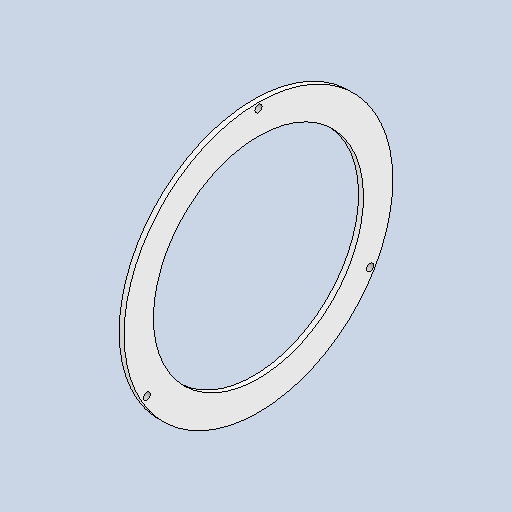
# Autodesk Inventor part: joint3_base_cover
Saved by Autodesk Inventor 2025.3 (Build 293356030, 356C)
## iProperties
Created: 2025-11-21
Part Number: joint3_base_cover
Material: PLA filament
Document SubType Name: Modeling
Designer: MSI
Mass: 17.2219 g
Surface Area: 134.924 cm^2
Volume: 14.3516 cm^3
Density: 1.2 g/cm^3
Appearance: 일반
Author: MSI
Autodesk Inventor part; units mm, degrees
ref_plane "YZ Plane" through (0, 0, 0) normal (1, 0, 0) x (0, 1, 0)
ref_plane "XZ Plane" through (0, 0, 0) normal (0, 1, 0) x (-1, 0, 0)
ref_plane "XY Plane" through (0, 0, 0) normal (0, 0, 1) x (1, 0, 0)
sketch "스케치1" plane through (0, 0, 0) normal (1, 0, 0) x (0, 1, 0)
  circle A0 centre (0, 0) radius 68.75
  circle A1 centre (0, 0) radius 53.75
  dimension "d0" = 137.5
  dimension "d1" = 15
  constraints: 2 centre point, 1 coincident
  measures "d0" diameter of A0
  measures "d1" radial gap between concentric circles of A0 A1
extrude "돌출1" add sketch "스케치1" along normal blind 2.5
sketch "스케치2" plane through (2.5, 0, 0) normal (1, 0, 0) x (0, 0, -1)
  line L0 (0, 0) -> (0, 66)
  dimension "d14" = 66
  constraints: 2 end point, 1 vertical
  measures "d14" distance of L0.start L0.end
hole "구멍1" at (2.5, 66, 0) direction (-1, 0, 0) diameter 3.6881 end through all thread size "M4.5x0.75" class "6H" standard "ISO Metric profile"
pattern_circular "원형 패턴1" count 3 over 360 about axis through (0, 0, 0) along (1, 0, 0) of "구멍1"
